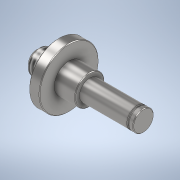
# Autodesk Inventor part: ParallelMecha_Gabel_Connection_JointShaft_Nadellager
Saved by Autodesk Inventor 2022 (Build 260153000, 153)
## iProperties
Created: 2022-07-21
Part Number: ParallelMecha_Gabel_Connection_JointShaft_Nadellager
Material: Edelstahl
Document SubType Name: Modeling
Designer: alexw
Density: 8 g/cm^3
Appearance: Halbpoliert
Mass: 24.4045 g
Surface Area: 19.8116 cm^2
Volume: 3.05056 cm^3
Flansch_Thickness: 3,500 mm
Gabel_FixationShaft_Contact_Thickness: 3,500 mm
Author: alexw
Autodesk Inventor part; units mm, degrees
ref_plane "YZ Plane" through (0, 0, 0) normal (1, 0, 0) x (0, 1, 0)
ref_plane "XZ Plane" through (0, 0, 0) normal (0, 1, 0) x (-1, 0, 0)
ref_plane "XY Plane" through (0, 0, 0) normal (0, 0, 1) x (1, 0, 0)
sketch "Skizze1" plane through (0, 0, 0) normal (0, 0, 1) x (1, 0, 0)
  line L0 (0, 0) -> (0, 10)
  line L1 (0, 10) -> (3.5, 10)
  line L2 (3.5, 10) -> (3.5, 5)
  line L3 (10.5, 3.5) -> (26.5, 3.5)
  line L4 (26.5, 3.5) -> (26.5, 3)
  line L5 (26.5, 3) -> (27.24, 3)
  line L6 (27.24, 3) -> (27.24, 3.5)
  line L7 (27.24, 3.5) -> (28.44, 3.5)
  line L8 (28.64, 3.3) -> (28.64, 0)
  line L9 (28.64, 0) -> (0, 0)
  line L10 (28.44, 3.5) -> (28.64, 3.3)
  line L11 (3.5, 5) -> (10.5, 5)
  line L12 (10.5, 5) -> (10.5, 3.5)
  line L13 (0, 4) -> (-7.5, 4)
  line L14 (-7.5, 4) -> (-7.5, 0)
  line L15 (-7.5, 0) -> (0, 0)
  point P0 (28.64, 3.5)
  dimension "d0" = 6
  dimension "d1" = 7
  dimension "d2" = 0.74
  dimension "d3" = 0.2
  dimension "d4" = 0.2
  dimension "d5" = 1.2
  dimension "d6" = 10
  dimension "d7" = 23
  dimension "d8" = 16
  dimension "d9" = 20
  dimension "Gabel_FixationShaft_Contact_Thickness" = 3.5
  dimension "d29" = 8
  dimension "d30" = 7.5
  constraints: 32 end point, 10 perpendicular, 5 point on line, 2 horizontal, 1 collinear, 1 vertical
  measures "d0" diameter of L5 L9
  measures "d1" diameter of L3 L9
  measures "d2" distance between parallel lines of L6 L4
  measures "d3" distance of L7.end point (28.64, 3.5)
  measures "d4" distance of L8.start point (28.64, 3.5)
  measures "d5" distance from line of L7.end L6
  measures "d6" diameter of L11 L9
  measures "d7" distance between parallel lines of L4 L2
  measures "d8" distance between parallel lines of L4 L12
  measures "d9" diameter of L1 L9
  measures "Gabel_FixationShaft_Contact_Thickness" distance between parallel lines of L0 L2
  measures "d29" diameter of L13 L15
  measures "d30" distance between parallel lines of L0 L14
revolve "Umdrehung1" add sketch "Skizze1" angle 360 about axis through (28.64, 0, 0) along (-1, 0, 0)
chamfer "Fase1" distance 0.2 angle 45 3 edges at (10.5, -5, 0) (3.5, -10, 0) (0, -10, 0)
chamfer "Fase2" distance 1.25 angle 45 1 edges at (-7.5, -4, 0)
thread "Gewinde1" size "M8x1.25" class "6g" standard "ANSI Metric M Profile" full length
equation "\"d3\" = d4"
